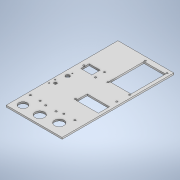
# Autodesk Inventor part: housing
Saved by Autodesk Inventor 2020 (Build 240168000, 168)
## iProperties
Created: 2021-12-06
Part Number: housing
Material: 일반
Document SubType Name: Modeling
Designer: d2h10s
Density: 1 g/cm^3
Appearance: 기본값
Author: d2h10s
Autodesk Inventor part; units mm, degrees
ref_plane "YZ Plane" through (0, 0, 0) normal (1, 0, 0) x (0, 1, 0)
ref_plane "XZ Plane" through (0, 0, 0) normal (0, 1, 0) x (-1, 0, 0)
ref_plane "XY Plane" through (0, 0, 0) normal (0, 0, 1) x (1, 0, 0)
sketch "스케치1" plane through (0, 0, 0) normal (0, 1, 0) x (-1, 0, 0)
  line L0 (50, 100) -> (-50, 100)
  line L1 (-50, 100) -> (-50, -100)
  line L2 (-50, -100) -> (50, -100)
  line L3 (50, -100) -> (50, 100)
  point P0 (0, 0)
  dimension "d0" = 100
  dimension "d1" = 200
  constraints: 8 end point, 2 parallel, 1 horizontal, 1 perpendicular
  measures "d0" distance of L2.end L1.end
  measures "d1" distance of L1.end L0.end
extrude "돌출1" add sketch "스케치1" along normal blind 3
sketch "스케치2" plane through (0, 0, 0) normal (0, -1, 0) x (1, 0, 0)
  circle A0 centre (25, 80) radius 8.5
  circle A1 centre (35, 62) radius 1.6
  circle A2 centre (15, 62) radius 1.6
  circle A3 centre (-5, 85) radius 8.5
  circle A4 centre (4.25, 65) radius 1.6
  circle A5 centre (-14.25, 65) radius 1.6
  circle A6 centre (-35, 85) radius 7.5
  circle A7 centre (-26.25, 63) radius 1.6
  circle A8 centre (-43.75, 63) radius 1.6
  line L0 (-50, 100) -> (50, 100) projected
  line L1 (-50, -100) -> (-50, 100) projected
  line L2 (45, 30) -> (5, 30)
  line L3 (5, 30) -> (5, 10)
  line L4 (5, 10) -> (45, 10)
  line L5 (45, 10) -> (45, 30)
  circle A9 centre (2.5, 28.5) radius 1.6
  circle A10 centre (43.5, -4.5) radius 1.6
  circle A11 centre (35, 20) radius 9.6 construction
  line L6 (7, 95) -> (-17, 95) construction
  line L7 (-17, 95) -> (-17, 61) construction
  line L8 (-17, 61) -> (7, 61) construction
  line L9 (7, 61) -> (7, 95) construction
  line L10 (38.25, 96) -> (11.75, 96) construction
  line L11 (11.75, 96) -> (11.75, 60) construction
  line L12 (11.75, 60) -> (38.25, 60) construction
  line L13 (38.25, 60) -> (38.25, 96) construction
  line L14 (-23.5, 95) -> (-46.5, 95) construction
  line L15 (-46.5, 95) -> (-46.5, 61) construction
  line L16 (-46.5, 61) -> (-23.5, 61) construction
  line L17 (-23.5, 61) -> (-23.5, 95) construction
  line L18 (46.5, -24) -> (3.5, -24) construction
  line L19 (3.5, -24) -> (3.5, -96) construction
  line L20 (3.5, -96) -> (46.5, -96) construction
  line L21 (46.5, -96) -> (46.5, -24) construction
  line L22 (46.5, -24) -> (3.5, -96) construction
  line L23 (3.5, -24) -> (46.5, -96) construction
  line L24 (44.5, -29) -> (5.5, -29)
  line L25 (5.5, -29) -> (5.5, -91)
  line L26 (5.5, -91) -> (44.5, -91)
  line L27 (44.5, -91) -> (44.5, -29)
  line L28 (44.5, -29) -> (5.5, -91) construction
  line L29 (5.5, -29) -> (44.5, -91) construction
  circle A12 centre (44.4, -93.5) radius 1.5
  circle A13 centre (5.6, -93.5) radius 1.5
  circle A14 centre (5.6, -26.5) radius 1.5
  circle A15 centre (44.4, -26.5) radius 1.5
  line L30 (-29, 29.5) -> (-48, 29.5) construction
  line L31 (-48, 29.5) -> (-48, 14.5) construction
  line L32 (-48, 14.5) -> (-29, 14.5) construction
  line L33 (-29, 14.5) -> (-29, 29.5) construction
  circle A16 centre (-40, 22) radius 2.5
  circle A17 centre (-45.9, 16.6) radius 1.1
  circle A18 centre (-45.9, 27.4) radius 1.1
  circle A19 centre (-40, 0) radius 8.5 construction
  circle A20 centre (-40, 0) radius 3.5
  line L34 (-39, -8) -> (-41, -8)
  line L35 (-41, -8) -> (-41, -9)
  line L36 (-41, -9) -> (-39, -9)
  line L37 (-39, -9) -> (-39, -8)
  line L38 (-39, -8) -> (-41, -9) construction
  line L39 (-41, -8) -> (-39, -9) construction
  line L40 (-20, -23.5) -> (-40, -23.5)
  line L41 (-40, -23.5) -> (-40, -38.5)
  line L42 (-40, -38.5) -> (-20, -38.5)
  line L43 (-20, -38.5) -> (-20, -23.5)
  line L44 (-20, -23.5) -> (-40, -38.5) construction
  line L45 (-40, -23.5) -> (-20, -38.5) construction
  line L46 (-3, -20) -> (-45, -20) construction
  line L47 (-45, -20) -> (-45, -42) construction
  line L48 (-45, -42) -> (-3, -42) construction
  line L49 (-3, -42) -> (-3, -20) construction
  line L50 (-3, -20) -> (-45, -42) construction
  line L51 (-45, -20) -> (-3, -42) construction
  circle A21 centre (-42, -31) radius 1.5
  circle A22 centre (-13, -39) radius 1.5
  circle A23 centre (-13, -23) radius 1.5
  point P0 (0, 0)
  point P1 (25, -60)
  point P2 (25, -60)
  point P3 (-40, -8.5)
  point P4 (-30, -31)
  point P5 (-24, -31)
  dimension "d9" = 17
  dimension "d10" = 3.2
  dimension "d11" = 3.2
  dimension "d12" = 18
  dimension "d13" = 20
  dimension "d14" = 10
  dimension "d15" = 18
  dimension "d16" = 17
  dimension "d17" = 20
  dimension "d18" = 18.5
  dimension "d19" = 9.25
  dimension "d20" = 20
  dimension "d21" = 3.2
  dimension "d22" = 3.2
  dimension "d23" = 15
  dimension "d24" = 3.2
  dimension "d25" = 22
  dimension "d26" = 3.2
  dimension "d27" = 17.5
  dimension "d28" = 8.75
  dimension "d29" = 22
  dimension "d30" = 20
  dimension "d31" = 15
  dimension "d32" = 15
  dimension "d33" = 15
  dimension "d34" = 30
  dimension "d35" = 30
  dimension "d36" = 40
  dimension "d37" = 20
  dimension "d38" = 55
  dimension "d39" = 70
  dimension "d40" = 3.2
  dimension "d41" = 3.2
  dimension "d42" = 33
  dimension "d43" = 41
  dimension "d44" = 19.2
  dimension "d45" = 10
  dimension "d46" = 10
  dimension "d47" = 24
  dimension "d48" = 34
  dimension "d49" = 12
  dimension "d50" = 10
  dimension "d51" = 26.5
  dimension "d52" = 36
  dimension "d53" = 16
  dimension "d54" = 13.25
  dimension "d55" = 23
  dimension "d56" = 34
  dimension "d57" = 11.5
  dimension "d58" = 10
  dimension "d59" = 8.5
  dimension "d60" = 32.5
  dimension "d65" = 43
  dimension "d66" = 72
  dimension "d67" = 39
  dimension "d68" = 62
  dimension "d69" = 3
  dimension "d70" = 2.1
  dimension "d71" = 2.5
  dimension "d72" = 3
  dimension "d73" = 2.5
  dimension "d74" = 2.1
  dimension "d75" = 3
  dimension "d76" = 2.5
  constraints: 100 end point, 24 centre point, 20 parallel, 11 midpoint, 10 horizontal, 10 perpendicular, 1 coincident
  measures "d9" diameter of A0
  measures "d10" diameter of A1
  measures "d11" diameter of A2
  measures "d12" vertical distance of A2.centre A0.centre
  measures "d13" distance of A1.centre A2.centre
  measures "d14" horizontal distance of A0.centre A2.centre
  measures "d15" vertical distance of A0.centre A1.centre
  measures "d16" diameter of A3
  measures "d17" vertical distance of A4.centre A3.centre
  measures "d18" distance of A4.centre A5.centre
  measures "d19" horizontal distance of A3.centre A4.centre
  measures "d20" vertical distance of A3.centre A5.centre
  measures "d21" diameter of A5
  measures "d22" diameter of A4
  measures "d23" diameter of A6
  measures "d24" diameter of A7
  measures "d25" vertical distance of A6.centre A7.centre
  measures "d26" diameter of A8
  measures "d27" distance of A7.centre A8.centre
  measures "d28" horizontal distance of A7.centre A6.centre
  measures "d29" vertical distance of A6.centre A8.centre
  measures "d30" distance from line of L0 A0.centre
  measures "d31" distance from line of L0 A3.centre
  measures "d32" distance from line of L0 A6.centre
  measures "d33" distance from line of L1 A6.centre
  measures "d34" distance of A6.centre A3.centre
  measures "d35" horizontal distance of A3.centre A0.centre
  measures "d36" distance of L4.end L3.end
  measures "d37" distance of L3.end L2.end
  measures "d38" distance between parallel lines of L1 L3
  measures "d39" distance between parallel lines of L0 L2
  measures "d40" diameter of A9
  measures "d41" diameter of A10
  measures "d42" vertical distance of A9.centre A10.centre
  measures "d43" horizontal distance of A9.centre A10.centre
  measures "d44" diameter of A11
  measures "d45" distance from line of L4 A11.centre
  measures "d46" distance from line of L5 A11.centre
  measures "d47" distance of L8.end L7.end
  measures "d48" distance of L7.end L6.end
  measures "d49" distance from line of A3.centre L9
  measures "d50" distance from line of L6 A3.centre
  measures "d51" distance of L12.end L11.end
  measures "d52" distance of L11.end L10.end
  measures "d53" distance from line of A0.centre L10
  measures "d54" distance from line of L13 A0.centre
  measures "d55" distance of L16.end L15.end
  measures "d56" distance of L15.end L14.end
  measures "d57" distance from line of A6.centre L17
  measures "d58" distance from line of L14 A6.centre
  measures "d59" vertical distance of A9.centre A11.centre
  measures "d60" horizontal distance of A11.centre A9.centre
  measures "d65" distance of L20.end L19.end
  measures "d66" distance of L19.end L18.end
  measures "d67" distance of L26.end L25.end
  measures "d68" distance of L25.end L24.end
  measures "d69" diameter of A12
  measures "d70" distance from line of L21 A12.centre
  measures "d71" distance from line of L20 A12.centre
  measures "d72" diameter of A13
  measures "d73" distance from line of L20 A13.centre
  measures "d74" distance from line of L19 A13.centre
  measures "d75" diameter of A14
  measures "d76" distance from line of L18 A14.centre
extrude "돌출2" cut sketch "스케치2" against normal through all
